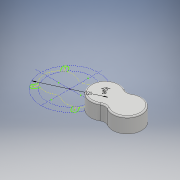
# Autodesk Inventor part: Gehaeuse_V3
Saved by Autodesk Inventor 2017 (Build 210142000, 142)
## iProperties
Created: 2019-05-23
Part Number: Gehaeuse_V3
Material: Generic
Document SubType Name: Modeling
Designer: Ole Simmering
Density: 1 g/cm^3
Appearance: Default
Author: Ole Simmering
Autodesk Inventor part; units mm, degrees
ref_plane "YZ Plane" through (0, 0, 0) normal (1, 0, 0) x (0, 1, 0)
ref_plane "XZ Plane" through (0, 0, 0) normal (0, 1, 0) x (-1, 0, 0)
ref_plane "XY Plane" through (0, 0, 0) normal (0, 0, 1) x (1, 0, 0)
sketch "Sketch1" plane through (0, 0, 0) normal (0, 0, 1) x (1, 0, 0)
  line L0 (-11.999, -0.0009) -> (209.001, -0.0009) construction
  circle A0 centre (47.001, -0.0009) radius 42.5 construction
  circle A1 centre (132.001, -0.0009) radius 42.5 construction
  circle A2 centre (47.001, -0.0009) radius 47.5625 construction
  circle A3 centre (132.001, -0.0009) radius 47.5625 construction
  arc A4 (82.1177, 32.0773) -> (-0.5615, -0.0019) centre (47.001, -0.0009) ccw
  arc A5 (179.5635, -0.0009) -> (96.8843, 32.0773) centre (132.001, -0.0009) ccw
  arc A6 (-0.5615, -0.0019) -> (82.1177, -32.079) centre (47.001, -0.0009) ccw
  arc A7 (96.8843, -32.079) -> (179.5635, -0.0009) centre (132.001, -0.0009) ccw
  arc A8 (75.7238, 47.5616) -> (-8.5615, -0.0015) centre (47.001, -0.0009) ccw
  arc A9 (187.5635, -0.0009) -> (103.2782, 47.5616) centre (132.001, -0.0009) ccw
  line L1 (47.001, 47.5616) -> (132.001, 47.5616) construction
  arc A10 (75.7238, 47.5616) -> (103.2782, 47.5616) centre (89.501, 70.3754) ccw
  arc A11 (-8.5615, -0.0015) -> (75.7238, -47.5634) centre (47.001, -0.0009) ccw
  arc A12 (103.2782, -47.5634) -> (187.5635, -0.0009) centre (132.001, -0.0009) ccw
  arc A13 (103.2782, -47.5634) -> (75.7238, -47.5634) centre (89.501, -70.3772) ccw
  arc A14 (82.1177, 32.0773) -> (96.8843, 32.0773) centre (89.501, 38.8217) ccw
  line L2 (82.1177, 32.0773) -> (96.8843, 32.0773) construction
  arc A15 (96.8843, -32.079) -> (82.1177, -32.079) centre (89.501, -38.8234) ccw
  point P0 (89.501, 21.3519)
  point P1 (46.9513, 55.5616)
  point P2 (132.0501, 55.5616)
  dimension "d5" = 221
  dimension "d6" = 85
  dimension "d7" = 85
  dimension "d8" = 85
  dimension "d9" = 95.125
  dimension "d10" = 95.125
  dimension "d12" = 8
  dimension "d20" = 10
  constraints: 36 point on circle, 16 centre point, 6 end point, 6 symmetric about line, 5 point on line, 5 tangent, 3 horizontal, 2 coincident, 2 concentric, 7 other
  measures "d5" distance of L0.start L0.end
  measures "d6" diameter of A0
  measures "d7" diameter of A1
  measures "d8" distance of A1.centre A0.centre
  measures "d9" diameter of A2
  measures "d10" diameter of A3
  measures "d12" radial gap between concentric circles of A4 A8
  measures "d20" radius of A14
extrude "Extrusion1" add sketch "Sketch1" along normal blind 50
sketch "Sketch2" plane through (0, 0, 50) normal (0, 0, 1) x (1, 0, 0)
  arc A0 (75.7238, 47.5616) -> (75.7238, -47.5634) centre (47.001, -0.0009) ccw projected
  arc A1 (75.7238, 47.5616) -> (103.2782, 47.5616) centre (89.501, 70.3754) ccw projected
  arc A2 (103.2782, -47.5634) -> (103.2782, 47.5616) centre (132.001, -0.0009) ccw projected
  arc A3 (103.2782, -47.5634) -> (75.7238, -47.5634) centre (89.501, -70.3772) ccw projected
  point P0 (0, 0)
extrude "Extrusion2" add sketch "Sketch2" along normal blind 8
fillet "Fillet1" radius 5 4 edges at (89.501, -43.7261, 58) (187.5635, -0.0009, 58) (89.501, 43.7243, 58) (-8.5615, -0.0009, 58)
sketch "Sketch4" plane through (0, 0, 0) normal (0, 0, -1) x (-1, 0, 0)
  arc A0 (75.7238, 47.5616) -> (103.2782, 47.5616) centre (89.501, 70.3754) ccw construction
  arc A1 (103.2782, -47.5634) -> (103.2782, 47.5616) centre (132.001, -0.0009) ccw construction
  arc A2 (103.2782, -47.5634) -> (75.7238, -47.5634) centre (89.501, -70.3772) ccw construction
  arc A3 (75.7238, 47.5616) -> (75.7238, -47.5634) centre (47.001, -0.0009) ccw construction
  circle A4 centre (89.501, -0.0009) radius 110.5 construction
  circle A5 centre (89.501, -0.0009) radius 85.5 construction
  line L0 (18.5679, 47.7354) -> (4.7605, 70.9167) construction
  line L1 (10.4408, 41.8386) -> (1.6244, 56.6404)
  arc A6 (5.0986, 70.3492) -> (1.6244, 56.6404) centre (10.2159, 61.7577) ccw
  line L2 (27.6237, 52.0732) -> (18.8073, 66.875)
  arc A7 (18.8073, 66.875) -> (5.0986, 70.3492) centre (10.2159, 61.7577) ccw
  line L3 (-70, -0.0009) -> (224, -0.0009) construction
  line L4 (89.501, -110.5009) -> (89.501, 124.0091) construction
  line L5 (160.434, 47.7354) -> (174.2414, 70.9167) construction
  line L6 (168.5612, 41.8386) -> (177.3775, 56.6404)
  arc A8 (177.3775, 56.6404) -> (173.9034, 70.3492) centre (168.7861, 61.7577) ccw
  arc A9 (173.9034, 70.3492) -> (160.1946, 66.875) centre (168.7861, 61.7577) ccw
  line L7 (151.3783, 52.0732) -> (160.1946, 66.875)
  arc A10 (103.2782, -47.5634) -> (75.7238, -47.5634) centre (89.501, -70.3772) ccw construction
  line L8 (18.5679, -47.7372) -> (4.7605, -70.9185) construction
  line L9 (10.4408, -41.8404) -> (1.6244, -56.6422)
  arc A11 (1.6244, -56.6422) -> (5.0986, -70.3509) centre (10.2159, -61.7595) ccw
  arc A12 (5.0986, -70.3509) -> (18.8073, -66.8768) centre (10.2159, -61.7595) ccw
  line L10 (27.6237, -52.075) -> (18.8073, -66.8768)
  line L11 (151.3783, -52.075) -> (160.1946, -66.8768)
  line L12 (168.5612, -41.8404) -> (177.3775, -56.6422)
  arc A13 (160.1946, -66.8768) -> (173.9034, -70.3509) centre (168.7861, -61.7595) ccw
  arc A14 (173.9034, -70.3509) -> (177.3775, -56.6422) centre (168.7861, -61.7595) ccw
  line L13 (160.434, -47.7372) -> (174.2414, -70.9185) construction
  dimension "d28" = 221
  dimension "d30" = 25
  dimension "d33" = 20
  constraints: 30 point on circle, 28 end point, 27 symmetric about line, 14 centre point, 6 point on line, 2 line through centre, 2 tangent, 1 coincident, 1 horizontal, 1 parallel, 1 vertical, 12 other
  measures "d28" diameter of A4
  measures "d33" distance between parallel lines of L2 L1
equation "\"d7\" = d6"
equation "\"d8\" = d6"
equation "\"d10\" = d9"
body "Solid1"
